Autodesk Fusion 360 part; units mm, degrees
(part 2 of 2)
equation "d42 = TowerY"
equation "d43 = TowerX"
equation "LidThickness = 0.5 in" comment "The thickness of the lid"
equation "d45 = LidThickness"
equation "d47 = LidThickness / 2"
equation "LidDrop = 0.5 in" comment "The length of the extruding fit on the lid"
equation "d49 = LidDrop"
equation "d51 = LidThickness / 2"
equation "d52 = LidDrop"
equation "d54 = LidThickness / 2"
equation "d55 = LidDrop"
equation "d57 = LidDrop"
equation "d59 = LidDrop"
equation "d61 = BaseX"
equation "d62 = BaseY"
equation "d63 = TowerX"
equation "d64 = TowerY"
equation "d65 = LidThickness"
equation "d67 = LidThickness / 2"
equation "d68 = -LidDrop"
equation "d70 = LidThickness / 2"
equation "d71 = -LidDrop"
equation "d73 = BaseThickness / 2"
equation "d74 = LidDrop"
equation "d76 = LidDrop"
equation "d78 = LidDrop"
equation "d82 = LidDrop"
equation "d84 = LidDrop"
equation "LidtoCutoffSide = ( BaseY - TowerY ) / 2" comment "How much the sides open"
equation "d87 = LidtoCutoffSide"
equation "d88 = LidtoCutoffSide"
equation "d96 = BaseThickness"
equation "d97 = BaseThickness / 2"
equation "d100 = BaseThickness"
equation "d101 = BaseThickness / 2"
equation "d104 = BaseThickness / 2"
equation "d105 = BaseThickness"
equation "d108 = BaseThickness"
equation "d109 = BaseThickness / 2"
equation "TowerDrop = 0.25 in" comment "the length of the extruding thing"
equation "SmallTopDroponTower = 0.5 in" comment "Does nothing but breaks stuff"
equation "d120 = SmallTopDroponTower"
equation "d125 = SmallTopDroponTower"
equation "d136 = TowerX - BaseDrop"
equation "d137 = TowerY - ( 2 * BaseDrop )"
equation "d138 = TowerThickness"
equation "d139 = TowerThickness"
equation "d140 = TowerThickness"
equation "d141 = TowerZ"
equation "d143 = howmuchtheliplengthis"
equation "howmuchtheliplengthis = 1 in"
equation "towerrabbit = 0.25 in" comment "how much the lip extrudes"
equation "d146 = TowerDrop"
equation "d147 = towerrabbit"
equation "d149 = howmuchtheliplengthis"
equation "d150 = TowerDrop"
equation "d151 = towerrabbit"
equation "d153 = howmuchtheliplengthis"
equation "d154 = TowerDrop"
equation "d155 = towerrabbit"
equation "d157 = howmuchtheliplengthis"
equation "d158 = TowerDrop"
equation "d159 = towerrabbit"
equation "d161 = towerrabbit"
equation "d163 = towerrabbit"
equation "insidetowerrabbit = 0.25 in" comment "depth"
equation "insidetowerdrop = 0.25 in" comment "length"
equation "d167 = TowerThickness / 2"
equation "d168 = insidetowerdrop"
equation "d169 = insidetowerrabbit"
equation "d171 = TowerThickness / 2"
equation "d172 = insidetowerdrop"
equation "d173 = insidetowerrabbit"
equation "d175 = TowerX - BaseDrop"
equation "d176 = TowerY - ( 2 * BaseDrop )"
equation "d177 = TowerThickness"
equation "d178 = TowerThickness"
equation "d179 = TowerThickness"
equation "d180 = TowerZ"
equation "d182 = TowerThickness / 2"
equation "d183 = insidetowerdrop"
equation "d184 = -insidetowerrabbit"
equation "d186 = TowerThickness / 2"
equation "d187 = insidetowerdrop"
equation "d188 = -insidetowerrabbit"
equation "d190 = TowerDrop"
equation "d191 = howmuchtheliplengthis"
equation "d192 = towerrabbit"
equation "d194 = howmuchtheliplengthis"
equation "d195 = TowerDrop"
equation "d196 = towerrabbit"
equation "d198 = TowerDrop"
equation "d199 = howmuchtheliplengthis"
equation "d200 = towerrabbit"
equation "d202 = howmuchtheliplengthis"
equation "d203 = TowerDrop"
equation "d204 = towerrabbit"
equation "d206 = towerrabbit"
equation "d208 = towerrabbit"
